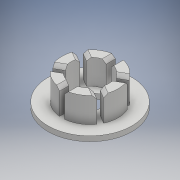
# Autodesk Inventor part: Compliance Adapter
Saved by Autodesk Inventor 2018 (Build 220112000, 112)
## iProperties
Created: 2018-01-21
Part Number: Compliance Adapter
Material: Generic
Document SubType Name: Modeling
Designer: Apple
Density: 1 g/cm^3
Appearance: Default
Author: Apple
Autodesk Inventor part; units mm, degrees
ref_plane "YZ Plane" through (0, 0, 0) normal (1, 0, 0) x (0, 1, 0)
ref_plane "XZ Plane" through (0, 0, 0) normal (0, 1, 0) x (-1, 0, 0)
ref_plane "XY Plane" through (0, 0, 0) normal (0, 0, 1) x (1, 0, 0)
sketch "Sketch1" plane through (0, 0, 0) normal (0, 0, 1) x (1, 0, 0)
  line L0 (-1.5, 18.1651) -> (1.5, 18.1651)
  line L1 (1.5, 18.1651) -> (1.5, 9.3755)
  line L2 (1.5, 9.3755) -> (-1.5, 9.3755)
  line L3 (-1.5, 9.3755) -> (-1.5, 18.1651)
  line L4 (-16.4814, 7.7835) -> (-14.9814, 10.3816)
  line L5 (-14.9814, 10.3816) -> (-7.3694, 5.9868)
  line L6 (-7.3694, 5.9868) -> (-8.8694, 3.3887)
  line L7 (-8.8694, 3.3887) -> (-16.4814, 7.7835)
  line L8 (-14.9814, -10.3816) -> (-16.4814, -7.7835)
  line L9 (-16.4814, -7.7835) -> (-8.8694, -3.3887)
  line L10 (-8.8694, -3.3887) -> (-7.3694, -5.9868)
  line L11 (-7.3694, -5.9868) -> (-14.9814, -10.3816)
  line L12 (1.5, -18.1651) -> (-1.5, -18.1651)
  line L13 (-1.5, -18.1651) -> (-1.5, -9.3755)
  line L14 (-1.5, -9.3755) -> (1.5, -9.3755)
  line L15 (1.5, -9.3755) -> (1.5, -18.1651)
  line L16 (16.4814, -7.7835) -> (14.9814, -10.3816)
  line L17 (14.9814, -10.3816) -> (7.3694, -5.9868)
  line L18 (7.3694, -5.9868) -> (8.8694, -3.3887)
  line L19 (8.8694, -3.3887) -> (16.4814, -7.7835)
  line L20 (14.9814, 10.3816) -> (16.4814, 7.7835)
  line L21 (16.4814, 7.7835) -> (8.8694, 3.3887)
  line L22 (8.8694, 3.3887) -> (7.3694, 5.9868)
  line L23 (7.3694, 5.9868) -> (14.9814, 10.3816)
  arc A0 (-1.5, 11.1496) -> (-8.9058, 6.8738) centre (0, 0) ccw
  arc A1 (-1.5, 16.6827) -> (-13.6976, 9.6404) centre (0, 0) ccw
  arc A2 (8.9058, 6.8738) -> (1.5, 11.1496) centre (0, 0) ccw
  arc A3 (13.6976, 9.6404) -> (1.5, 16.6827) centre (0, 0) ccw
  arc A4 (10.4058, -4.2757) -> (10.4058, 4.2757) centre (0, 0) ccw
  arc A5 (15.1976, -7.0423) -> (15.1976, 7.0423) centre (0, 0) ccw
  arc A6 (1.5, -11.1496) -> (8.9058, -6.8738) centre (0, 0) ccw
  arc A7 (-10.4058, 4.2757) -> (-10.4058, -4.2757) centre (0, 0) ccw
  arc A8 (-8.9058, -6.8738) -> (-1.5, -11.1496) centre (0, 0) ccw
  arc A9 (-15.1976, 7.0423) -> (-15.1976, -7.0423) centre (0, 0) ccw
  arc A10 (-13.6976, -9.6404) -> (-1.5, -16.6827) centre (0, 0) ccw
  arc A11 (1.5, -16.6827) -> (13.6976, -9.6404) centre (0, 0) ccw
  point P0 (0, 9.3755)
  point P1 (-8.1194, 4.6878)
  point P2 (-8.1194, -4.6878)
  point P3 (0, -9.3755)
  point P4 (8.1194, -4.6878)
  point P5 (8.1194, 4.6878)
  dimension "d16" = 3
  dimension "d19" = 360
  constraints: 48 end point, 24 point on circle, 24 point on line, 12 centre point, 2 parallel, 1 coincident, 1 horizontal, 1 midpoint, 1 perpendicular, 1 vertical alignment, 55 other
  measures "d16" distance of L0.start L0.end
extrude "Extrusion3" add sketch "Sketch1" along normal blind 15 contours L3 A0 L5 A1 | A3 L23 A2 L1 | L7 A7 L9 A9 | A5 L19 A4 L21 | L11 A8 L13 A10 | A11 L15 A6 L17
chamfer "Chamfer1" distance 2 angle 45 12 edges at (-1.5, 13.9161, 15) (1.5, 13.9161, 15) (11.3017, 8.2571, 15) (12.8017, 5.659, 15) (12.8017, -5.659, 15) (11.3017, -8.2571, 15) (1.5, -13.9161, 15) (-1.5, -13.9161, 15) (-11.3017, -8.2571, 15) (-12.8017, -5.659, 15) (-12.8017, 5.659, 15) (-11.3017, 8.2571, 15)
sketch "Sketch4" plane through (0, 0, 0) normal (0, 0, -1) x (-1, 0, 0)
  circle A0 centre (0, 0) radius 25
  line L0 (6.45, -3.7239) -> (0, -7.4478)
  line L1 (0, -7.4478) -> (-6.45, -3.7239)
  line L2 (-6.45, -3.7239) -> (-6.45, 3.7239)
  line L3 (-6.45, 3.7239) -> (0, 7.4478)
  line L4 (0, 7.4478) -> (6.45, 3.7239)
  line L5 (6.45, 3.7239) -> (6.45, -3.7239)
  dimension "d26" = 50
  dimension "d27" = 12.9
  constraints: 12 end point, 2 coincident, 1 centre point, 13 other
  measures "d26" diameter of A0
  measures "d27" distance between parallel lines of L2 L5
extrude "Extrusion4" add sketch "Sketch4" along normal blind 3
body "Solid2"
